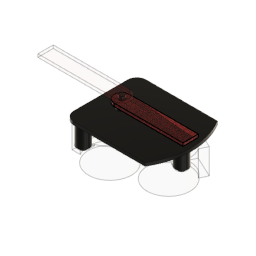
Clock_Assembly (1) (Autodesk Fusion 360 archive; units mm, degrees)
design "Movement"
description: Spur Gear; Module: 1.000000; Num Teeth: 20; Pressure Angle: 20.000000; Backlash: 0.10 mm
Autodesk Fusion 360 part; units mm, degrees
cylinder "CylinderPrimitive1" add diameter 28 height 19 placed x (1, 0, 0) y (0, 1, 0) z (0, 0, 1) at (0, 0, 0) makes body 1 in component "Motor"
sketch "Sketch2" plane through (0, 0, 19) normal (0, 0, 1) x (-1, 0, 0) in component "Motor"
  circle A0 centre (0, 0) radius 14
  line L0 (3.5, -13.5554) -> (3.5, -17.5)
  line L1 (-3.5, -13.5554) -> (-3.5, -17.5)
  line L2 (0, 0) -> (0, -14) construction
  line L3 (3.5, -17.5) -> (-3.5, -17.5) construction
  arc A1 (-3.5, -17.5) -> (3.5, -17.5) centre (0, -17.5) ccw
  circle A2 centre (0, -17.5) radius 2.05
  line L4 (0, 0) -> (-14, 0) construction
  arc A3 (3.5, 17.5) -> (-3.5, 17.5) centre (0, 17.5) ccw
  circle A4 centre (0, 17.5) radius 2.05
  line L5 (3.5, 13.5554) -> (3.5, 17.5)
  line L6 (-3.5, 13.5554) -> (-3.5, 17.5)
  circle A5 centre (-7.8, 0) radius 4.5
  circle A6 centre (-7.8, 0) radius 2.45
  line L7 (-7.8, 0) -> (-7.8, -2.45) construction
  line L8 (-9.3, -1.9371) -> (-9.3, 1.9371)
  line L9 (-6.3, -1.9371) -> (-6.3, 1.9371)
  line L10 (11.8216, -7.5) -> (17.2, -7.5)
  line L11 (17.2, -7.5) -> (17.2, 7.5)
  line L12 (17.2, 7.5) -> (11.8216, 7.5)
  line L13 (14, 0) -> (17.2, 0) construction
  dimension "d3" = 3.5
  dimension "d4" = 3.5
  dimension "d5" = 7
  dimension "d6" = 4.1
  dimension "d7" = 9
  dimension "d9" = 1.7
  dimension "d10" = 4.9
  dimension "d11" = 1.5
  dimension "d12" = 1.5
  dimension "d23" = 7.5
  dimension "d24" = 7.5
  dimension "d25" = 3.2
  constraint coincident A0 L0.start
  constraint vertical L0
  constraint coincident A0 L1.start
  constraint vertical L1
  constraint coincident A0.centre L2.start
  constraint coincident A0 L2.end
  constraint vertical L2
  constraint horizontal L3
  constraint midpoint L3 A1.centre
  constraint concentric A1 A2
  constraint coincident A0 L4.end
  constraint perpendicular L2 L4
  constraint symmetric L0.start L4 L5.start
  constraint symmetric L0.end L4 A3.start
  constraint symmetric L1.start L4 L6.start
  constraint symmetric L1.end L4 A3.end
  constraint symmetric A1 L4 A3
  constraint symmetric A2 L4 A4
  constraint coincident L4 A5.centre
  constraint concentric A5 A6
  constraint coincident A5.centre A6.centre
  constraint coincident A6 L7.end
  constraint perpendicular L4 L7
  constraint coincident A6 L8.start
  constraint coincident A6 L8.end
  constraint vertical L8
  constraint coincident A6 L9.start
  constraint coincident A6 L9.end
  constraint parallel L8 L9
  constraint coincident A0 L10.start
  constraint horizontal L10
  constraint perpendicular L10 L11
  constraint coincident A0 L12.end
  constraint perpendicular L11 L12
  constraint coincident A0 L13.start
  constraint coincident L11 L13.end
  constraint perpendicular L11 L13
  constraint collinear L4 L13
  measures "d3" distance of L0 L2
  measures "d4" distance of L1 L2
  measures "d5" distance of L2.end A1
  measures "d6" diameter of A2
  measures "d7" diameter of A5
  measures "d9" distance of L4.end A5
  measures "d10" diameter of A6
  measures "d11" distance of L7 L8
  measures "d12" distance of L7 L9
  measures "d23" distance of L12 L13
  measures "d24" distance of L10 L13
  measures "d25" distance of A0 L11
extrude "Extrude1" add sketch "Sketch2" against normal blind 0.85 contours A0 A3 L5 L6 | A0 L0 L1 A1 bodies 1 in component "Motor"
extrude "Extrude2" add sketch "Sketch2" along normal blind 1.7 contours A5 | A6 L9 | A6 L8 L9 | A6 L8 bodies 1 in component "Motor"
extrude "Extrude3" add sketch "Sketch2" along normal blind 2.25 from surface at 1.7 contours A6 L9 | A6 L8 L9 | A6 L8 bodies 1 in component "Motor"
extrude "Extrude4" add sketch "Sketch2" along normal blind 10 contours A6 L8 L9 bodies 1 in component "Motor"
extrude "Extrude5" add sketch "Sketch2" against normal blind 16.5 contours A0 L10 L11 L12 bodies 1 in component "Motor"
sketch "Sketch1" plane through (0, 0, 29) normal (0, 0, 1) x (-1, 0, 0) in component "Minute Hand"
  arc A0 (-9.3, -1.9371) -> (-6.3, -1.9371) centre (-7.8, 0) ccw construction
  line L0 (-6.3, -1.9371) -> (-6.3, 1.9371) construction
  arc A1 (-6.3, 1.9371) -> (-9.3, 1.9371) centre (-7.8, 0) ccw construction
  line L1 (-9.3, 1.9371) -> (-9.3, -1.9371)
  line L2 (-6.3, 1.9371) -> (-6.3, -1.9371) construction
  arc A2 (-6.3, -1.9371) -> (-6.3, 1.9371) centre (-7.8, 0) ccw construction
  line L3 (-9.3, -1.9371) -> (-9.3, 1.9371) construction
  arc A3 (-9.3, 1.9371) -> (-9.3, -1.9371) centre (-7.8, 0) ccw construction
  arc A4 (-5.0755, -3.5185) -> (-5.0755, 3.5185) centre (-7.8, 0) ccw
  arc A5 (-5.0755, 3.5185) -> (-10.5245, 3.5185) centre (-7.8, 0) ccw
  arc A6 (-10.5245, 3.5185) -> (-10.5245, -3.5185) centre (-7.8, 0) ccw
  arc A7 (-10.5245, -3.5185) -> (-5.0755, -3.5185) centre (-7.8, 0) ccw
  arc A8 (-6.2, 1.9856) -> (-9.4, 1.9856) centre (-7.8, 0) ccw
  line L4 (-9.4, -1.9856) -> (-9.4, 1.9856)
  arc A9 (-9.4, -1.9856) -> (-6.2, -1.9856) centre (-7.8, 0) ccw
  line L5 (-6.2, -1.9856) -> (-6.2, 1.9856)
  circle A10 centre (-7.8, 0) radius 1.6
  dimension "d28" = 2
  dimension "d29" = 0.1
  dimension "d32" = 3.2
  constraint concentric A3 A10
  measures "d32" diameter of A10
extrude "Extrude1'" add sketch "Sketch1" against normal up to surface (5.05 mm away) separate body makes body 2 in component "Minute Hand"
extrude "Extrude3'" add sketch "Sketch1" along normal blind 1 contours L1 A10 | A8 L4 L5 A10 | L1 A10 | L4 A9 L5 A10 | A4 A5 A6 A7 bodies 2 in component "Minute Hand"
extrude "Extrude2'" add sketch "Sketch1" along normal blind 12.5 from surface at 1 contours L1 A10 | L1 A10 bodies 2 in component "Minute Hand"
sketch "Sketch1 (2)" plane through (0, 0, 0) normal (0, 0, 1) x (1, 0, 0) in component "Hour Hand"
  circle A0 centre (0, 0) radius 8.7492
extrude "Extrude1''" add sketch "Sketch1 (2)" along normal blind 3 separate body makes body 3 in component "Hour Hand"
sketch "Sketch2 (2)" plane through (0, 0, 0) normal (0, 0, 1) x (1, 0, 0) in component "Hour Hand"
  spline S0 degree 5 poles (9.3581, -0.8534) (9.3628, -0.8538) (9.3721, -0.8546) (9.3861, -0.8553) (9.4048, -0.8555) (9.4282, -0.8549) (9.4516, -0.8535) (9.4751, -0.8518) (9.4986, -0.8498) (9.5221, -0.8476) (9.5456, -0.8452) (9.5692, -0.8427) (9.5927, -0.8398) (9.6163, -0.8366) (9.6398, -0.8331) (9.6634, -0.8293) (9.687, -0.8252) (9.7106, -0.8208) (9.7342, -0.8163) (9.7577, -0.8116) (9.7813, -0.8067) (9.8049, -0.8015) (9.8285, -0.7962) (9.8521, -0.7907) (9.8757, -0.7849) (9.8993, -0.779) (9.9228, -0.7729) (9.9464, -0.7665) (9.97, -0.76) (9.9935, -0.7533) (10.0171, -0.7465) (10.0407, -0.7394) (10.0642, -0.7322) (10.0877, -0.7249) (10.1113, -0.7173) (10.1348, -0.7096) (10.1583, -0.7017) (10.1818, -0.6937) (10.2053, -0.6855) (10.2288, -0.6771) (10.2523, -0.6686) (10.2758, -0.6599) (10.2992, -0.6511) (10.3227, -0.6421) (10.3461, -0.633) (10.3695, -0.6237) (10.3929, -0.6143) (10.4163, -0.6047) (10.4397, -0.5949) (10.463, -0.5851) (10.4864, -0.5751) (10.5097, -0.5649) (10.533, -0.5546) (10.5563, -0.5441) (10.5796, -0.5336) (10.6029, -0.5228) (10.6261, -0.512) (10.6493, -0.501) (10.6726, -0.4898) (10.6957, -0.4785) (10.7189, -0.4671) (10.7421, -0.4556) (10.7652, -0.4439) (10.7883, -0.4321) (10.8114, -0.4201) (10.8345, -0.4081) (10.8575, -0.3959) (10.8806, -0.3835) (10.9036, -0.3711) (10.9265, -0.3585) (10.9495, -0.3458) (10.9679, -0.3355) (10.9816, -0.3277) (10.9908, -0.3225) (10.9953, -0.3199) knots 0 0 0 0 0 0 0.01428571 0.02857143 0.04285714 0.05714286 0.07142857 0.08571429 0.1 0.11428571 0.12857143 0.14285714 0.15714286 0.17142857 0.18571429 0.2 0.21428571 0.22857143 0.24285714 0.25714286 0.27142857 0.28571429 0.3 0.31428571 0.32857143 0.34285714 0.35714286 0.37142857 0.38571429 0.4 0.41428571 0.42857143 0.44285714 0.45714286 0.47142857 0.48571429 0.5 0.51428571 0.52857143 0.54285714 0.55714286 0.57142857 0.58571429 0.6 0.61428571 0.62857143 0.64285714 0.65714286 0.67142857 0.68571429 0.7 0.71428571 0.72857143 0.74285714 0.75714286 0.77142857 0.78571429 0.8 0.81428571 0.82857143 0.84285714 0.85714286 0.87142857 0.88571429 0.9 0.91428571 0.92857143 0.94285714 0.95714286 0.97142857 0.98571429 1 1 1 1 1 1
  spline S1 degree 5 poles (9.3581, 0.8534) (9.3628, 0.8538) (9.3721, 0.8546) (9.3861, 0.8553) (9.4048, 0.8555) (9.4282, 0.8549) (9.4516, 0.8535) (9.4751, 0.8518) (9.4986, 0.8498) (9.5221, 0.8476) (9.5456, 0.8452) (9.5692, 0.8427) (9.5927, 0.8398) (9.6163, 0.8366) (9.6398, 0.8331) (9.6634, 0.8293) (9.687, 0.8252) (9.7106, 0.8208) (9.7342, 0.8163) (9.7577, 0.8116) (9.7813, 0.8067) (9.8049, 0.8015) (9.8285, 0.7962) (9.8521, 0.7907) (9.8757, 0.7849) (9.8993, 0.779) (9.9228, 0.7729) (9.9464, 0.7665) (9.97, 0.76) (9.9935, 0.7533) (10.0171, 0.7465) (10.0407, 0.7394) (10.0642, 0.7322) (10.0877, 0.7249) (10.1113, 0.7173) (10.1348, 0.7096) (10.1583, 0.7017) (10.1818, 0.6937) (10.2053, 0.6855) (10.2288, 0.6771) (10.2523, 0.6686) (10.2758, 0.6599) (10.2992, 0.6511) (10.3227, 0.6421) (10.3461, 0.633) (10.3695, 0.6237) (10.3929, 0.6143) (10.4163, 0.6047) (10.4397, 0.5949) (10.463, 0.5851) (10.4864, 0.5751) (10.5097, 0.5649) (10.533, 0.5546) (10.5563, 0.5441) (10.5796, 0.5336) (10.6029, 0.5228) (10.6261, 0.512) (10.6493, 0.501) (10.6726, 0.4898) (10.6957, 0.4785) (10.7189, 0.4671) (10.7421, 0.4556) (10.7652, 0.4439) (10.7883, 0.4321) (10.8114, 0.4201) (10.8345, 0.4081) (10.8575, 0.3959) (10.8806, 0.3835) (10.9036, 0.3711) (10.9265, 0.3585) (10.9495, 0.3458) (10.9679, 0.3355) (10.9816, 0.3277) (10.9908, 0.3225) (10.9953, 0.3199) knots 0 0 0 0 0 0 0.01428571 0.02857143 0.04285714 0.05714286 0.07142857 0.08571429 0.1 0.11428571 0.12857143 0.14285714 0.15714286 0.17142857 0.18571429 0.2 0.21428571 0.22857143 0.24285714 0.25714286 0.27142857 0.28571429 0.3 0.31428571 0.32857143 0.34285714 0.35714286 0.37142857 0.38571429 0.4 0.41428571 0.42857143 0.44285714 0.45714286 0.47142857 0.48571429 0.5 0.51428571 0.52857143 0.54285714 0.55714286 0.57142857 0.58571429 0.6 0.61428571 0.62857143 0.64285714 0.65714286 0.67142857 0.68571429 0.7 0.71428571 0.72857143 0.74285714 0.75714286 0.77142857 0.78571429 0.8 0.81428571 0.82857143 0.84285714 0.85714286 0.87142857 0.88571429 0.9 0.91428571 0.92857143 0.94285714 0.95714286 0.97142857 0.98571429 1 1 1 1 1 1
  arc A0 (10.9953, -0.3199) -> (10.9953, 0.3199) centre (0, 0) ccw
  line L0 (8.7031, -0.7946) -> (9.3581, -0.8534)
  line L1 (8.7031, 0.7946) -> (9.3581, 0.8534)
  line L2 (8.7031, -0.7946) -> (8.7031, 0.7946)
  point P0 (9.4732, -0.8519)
  point P1 (9.5892, -0.8402)
  point P2 (9.7057, -0.8217)
  point P3 (9.8226, -0.7975)
  point P4 (9.9398, -0.7683)
  point P5 (10.0572, -0.7344)
  point P6 (10.1747, -0.6961)
  point P7 (10.2922, -0.6537)
  point P8 (10.4098, -0.6073)
  point P9 (10.5272, -0.5571)
  point P10 (10.6446, -0.5032)
  point P11 (10.7618, -0.4456)
  point P12 (10.8787, -0.3845)
  point P13 (9.4732, 0.8519)
  point P14 (9.5892, 0.8402)
  point P15 (9.7057, 0.8217)
  point P16 (9.8226, 0.7975)
  point P17 (9.9398, 0.7683)
  point P18 (10.0572, 0.7344)
  point P19 (10.1747, 0.6961)
  point P20 (10.2922, 0.6537)
  point P21 (10.4098, 0.6073)
  point P22 (10.5272, 0.5571)
  point P23 (10.6446, 0.5032)
  point P24 (10.7618, 0.4456)
  point P25 (10.8787, 0.3845)
extrude "Extrude2''" add sketch "Sketch2 (2)" along normal blind 3 bodies 3 in component "Hour Hand"
fillet "Fillet1" radius 0.5 2 edges at (8.713, -0.7955, 1.5) (8.713, 0.7955, 1.5) on bodies 3 in component "Hour Hand"
pattern_circular "C-Pattern1" count 20 over 360 about axis through (0, 0, 0) along (0, 0, 1) of "Extrude2''", "Fillet1" in component "Hour Hand"
sketch "Sketch3" plane through (0, 0, 0) normal (0, 0, 1) x (1, 0, 0) in component "Hour Hand"
  circle A0 centre (0, 0) radius 10 construction
sketch "Sketch4" plane through (0, 0, 3) normal (0, 0, 1) x (-1, 0, 0) in component "Hour Hand"
  circle A0 centre (0, 0) radius 1.75
  circle A1 centre (0, 0) radius 3
  dimension "d56" = 3.5
  dimension "d57" = 6
  constraint coincident A0.centre A1.centre
  measures "d56" diameter of A0
  measures "d57" diameter of A1
extrude "Extrude3''" cut sketch "Sketch4" against normal through all contours A0 bodies 3 in component "Hour Hand"
extrude "Extrude4'" add sketch "Sketch4" along normal blind 6.5 bodies 3 in component "Hour Hand"
sketch "Sketch1 (3)" plane through (0, 0, 0) normal (0, 0, 1) x (1, 0, 0) in component "Spur Gear (20 teeth)"
  circle A0 centre (0, 0) radius 8.7492
extrude "Extrude1'''" add sketch "Sketch1 (3)" along normal blind 3 separate body makes body 4 in component "Spur Gear (20 teeth)"
sketch "Sketch2 (3)" plane through (0, 0, 0) normal (0, 0, 1) x (1, 0, 0) in component "Spur Gear (20 teeth)"
  spline S0 degree 5 poles (9.3581, -0.8534) (9.3628, -0.8538) (9.3721, -0.8546) (9.3861, -0.8553) (9.4048, -0.8555) (9.4282, -0.8549) (9.4516, -0.8535) (9.4751, -0.8518) (9.4986, -0.8498) (9.5221, -0.8476) (9.5456, -0.8452) (9.5692, -0.8427) (9.5927, -0.8398) (9.6163, -0.8366) (9.6398, -0.8331) (9.6634, -0.8293) (9.687, -0.8252) (9.7106, -0.8208) (9.7342, -0.8163) (9.7577, -0.8116) (9.7813, -0.8067) (9.8049, -0.8015) (9.8285, -0.7962) (9.8521, -0.7907) (9.8757, -0.7849) (9.8993, -0.779) (9.9228, -0.7729) (9.9464, -0.7665) (9.97, -0.76) (9.9935, -0.7533) (10.0171, -0.7465) (10.0407, -0.7394) (10.0642, -0.7322) (10.0877, -0.7249) (10.1113, -0.7173) (10.1348, -0.7096) (10.1583, -0.7017) (10.1818, -0.6937) (10.2053, -0.6855) (10.2288, -0.6771) (10.2523, -0.6686) (10.2758, -0.6599) (10.2992, -0.6511) (10.3227, -0.6421) (10.3461, -0.633) (10.3695, -0.6237) (10.3929, -0.6143) (10.4163, -0.6047) (10.4397, -0.5949) (10.463, -0.5851) (10.4864, -0.5751) (10.5097, -0.5649) (10.533, -0.5546) (10.5563, -0.5441) (10.5796, -0.5336) (10.6029, -0.5228) (10.6261, -0.512) (10.6493, -0.501) (10.6726, -0.4898) (10.6957, -0.4785) (10.7189, -0.4671) (10.7421, -0.4556) (10.7652, -0.4439) (10.7883, -0.4321) (10.8114, -0.4201) (10.8345, -0.4081) (10.8575, -0.3959) (10.8806, -0.3835) (10.9036, -0.3711) (10.9265, -0.3585) (10.9495, -0.3458) (10.9679, -0.3355) (10.9816, -0.3277) (10.9908, -0.3225) (10.9953, -0.3199) knots 0 0 0 0 0 0 0.01428571 0.02857143 0.04285714 0.05714286 0.07142857 0.08571429 0.1 0.11428571 0.12857143 0.14285714 0.15714286 0.17142857 0.18571429 0.2 0.21428571 0.22857143 0.24285714 0.25714286 0.27142857 0.28571429 0.3 0.31428571 0.32857143 0.34285714 0.35714286 0.37142857 0.38571429 0.4 0.41428571 0.42857143 0.44285714 0.45714286 0.47142857 0.48571429 0.5 0.51428571 0.52857143 0.54285714 0.55714286 0.57142857 0.58571429 0.6 0.61428571 0.62857143 0.64285714 0.65714286 0.67142857 0.68571429 0.7 0.71428571 0.72857143 0.74285714 0.75714286 0.77142857 0.78571429 0.8 0.81428571 0.82857143 0.84285714 0.85714286 0.87142857 0.88571429 0.9 0.91428571 0.92857143 0.94285714 0.95714286 0.97142857 0.98571429 1 1 1 1 1 1
  spline S1 degree 5 poles (9.3581, 0.8534) (9.3628, 0.8538) (9.3721, 0.8546) (9.3861, 0.8553) (9.4048, 0.8555) (9.4282, 0.8549) (9.4516, 0.8535) (9.4751, 0.8518) (9.4986, 0.8498) (9.5221, 0.8476) (9.5456, 0.8452) (9.5692, 0.8427) (9.5927, 0.8398) (9.6163, 0.8366) (9.6398, 0.8331) (9.6634, 0.8293) (9.687, 0.8252) (9.7106, 0.8208) (9.7342, 0.8163) (9.7577, 0.8116) (9.7813, 0.8067) (9.8049, 0.8015) (9.8285, 0.7962) (9.8521, 0.7907) (9.8757, 0.7849) (9.8993, 0.779) (9.9228, 0.7729) (9.9464, 0.7665) (9.97, 0.76) (9.9935, 0.7533) (10.0171, 0.7465) (10.0407, 0.7394) (10.0642, 0.7322) (10.0877, 0.7249) (10.1113, 0.7173) (10.1348, 0.7096) (10.1583, 0.7017) (10.1818, 0.6937) (10.2053, 0.6855) (10.2288, 0.6771) (10.2523, 0.6686) (10.2758, 0.6599) (10.2992, 0.6511) (10.3227, 0.6421) (10.3461, 0.633) (10.3695, 0.6237) (10.3929, 0.6143) (10.4163, 0.6047) (10.4397, 0.5949) (10.463, 0.5851) (10.4864, 0.5751) (10.5097, 0.5649) (10.533, 0.5546) (10.5563, 0.5441) (10.5796, 0.5336) (10.6029, 0.5228) (10.6261, 0.512) (10.6493, 0.501) (10.6726, 0.4898) (10.6957, 0.4785) (10.7189, 0.4671) (10.7421, 0.4556) (10.7652, 0.4439) (10.7883, 0.4321) (10.8114, 0.4201) (10.8345, 0.4081) (10.8575, 0.3959) (10.8806, 0.3835) (10.9036, 0.3711) (10.9265, 0.3585) (10.9495, 0.3458) (10.9679, 0.3355) (10.9816, 0.3277) (10.9908, 0.3225) (10.9953, 0.3199) knots 0 0 0 0 0 0 0.01428571 0.02857143 0.04285714 0.05714286 0.07142857 0.08571429 0.1 0.11428571 0.12857143 0.14285714 0.15714286 0.17142857 0.18571429 0.2 0.21428571 0.22857143 0.24285714 0.25714286 0.27142857 0.28571429 0.3 0.31428571 0.32857143 0.34285714 0.35714286 0.37142857 0.38571429 0.4 0.41428571 0.42857143 0.44285714 0.45714286 0.47142857 0.48571429 0.5 0.51428571 0.52857143 0.54285714 0.55714286 0.57142857 0.58571429 0.6 0.61428571 0.62857143 0.64285714 0.65714286 0.67142857 0.68571429 0.7 0.71428571 0.72857143 0.74285714 0.75714286 0.77142857 0.78571429 0.8 0.81428571 0.82857143 0.84285714 0.85714286 0.87142857 0.88571429 0.9 0.91428571 0.92857143 0.94285714 0.95714286 0.97142857 0.98571429 1 1 1 1 1 1
  arc A0 (10.9953, -0.3199) -> (10.9953, 0.3199) centre (0, 0) ccw
  line L0 (8.7031, -0.7946) -> (9.3581, -0.8534)
  line L1 (8.7031, 0.7946) -> (9.3581, 0.8534)
  line L2 (8.7031, -0.7946) -> (8.7031, 0.7946)
  point P0 (9.4732, -0.8519)
  point P1 (9.5892, -0.8402)
  point P2 (9.7057, -0.8217)
  point P3 (9.8226, -0.7975)
  point P4 (9.9398, -0.7683)
  point P5 (10.0572, -0.7344)
  point P6 (10.1747, -0.6961)
  point P7 (10.2922, -0.6537)
  point P8 (10.4098, -0.6073)
  point P9 (10.5272, -0.5571)
  point P10 (10.6446, -0.5032)
  point P11 (10.7618, -0.4456)
  point P12 (10.8787, -0.3845)
  point P13 (9.4732, 0.8519)
  point P14 (9.5892, 0.8402)
  point P15 (9.7057, 0.8217)
  point P16 (9.8226, 0.7975)
  point P17 (9.9398, 0.7683)
  point P18 (10.0572, 0.7344)
  point P19 (10.1747, 0.6961)
  point P20 (10.2922, 0.6537)
  point P21 (10.4098, 0.6073)
  point P22 (10.5272, 0.5571)
  point P23 (10.6446, 0.5032)
  point P24 (10.7618, 0.4456)
  point P25 (10.8787, 0.3845)
extrude "Extrude2'''" add sketch "Sketch2 (3)" along normal blind 3 bodies 4 in component "Spur Gear (20 teeth)"
fillet "Fillet1'" radius 0.5 2 edges at (8.713, -0.7955, 1.5) (8.713, 0.7955, 1.5) on bodies 4 in component "Spur Gear (20 teeth)"
pattern_circular "C-Pattern1'" count 20 over 360 about axis through (0, 0, 0) along (0, 0, 1) of "Extrude2'''", "Fillet1'" in component "Spur Gear (20 teeth)"
sketch "Sketch3 (2)" plane through (0, 0, 0) normal (0, 0, 1) x (1, 0, 0) in component "Spur Gear (20 teeth)"
  circle A0 centre (0, 0) radius 10 construction
sketch "Sketch4 (2)" plane through (0, 0, 3) normal (0, 0, 1) x (-1, 0, 0) in component "Spur Gear (20 teeth)"
  arc A0 (2.3896, -0.5408) -> (1.1217, 2.1781) centre (0, 0) ccw construction
  line L0 (2.3896, -0.5408) -> (-1.1217, -2.1781) construction
  arc A1 (-2.3896, 0.5408) -> (-1.1217, -2.1781) centre (0, 0) ccw construction
  line L1 (-2.3896, 0.5408) -> (1.1217, 2.1781) construction
  arc A2 (1.1217, 2.1781) -> (-2.3896, 0.5408) centre (0, 0) ccw construction
  arc A3 (-1.1217, -2.1781) -> (2.3896, -0.5408) centre (0, 0) ccw construction
  arc A4 (2.0374, 3.9562) -> (-4.3402, 0.9823) centre (0, 0) ccw
  arc A5 (-4.3402, 0.9823) -> (-2.0374, -3.9562) centre (0, 0) ccw
  arc A6 (-2.0374, -3.9562) -> (4.3402, -0.9823) centre (0, 0) ccw
  arc A7 (4.3402, -0.9823) -> (2.0374, 3.9562) centre (0, 0) ccw
  line L2 (-2.4757, 0.611) -> (1.1234, 2.2892)
  arc A8 (2.4757, -0.611) -> (1.1234, 2.2892) centre (0, 0) ccw
  line L3 (2.4757, -0.611) -> (-1.1234, -2.2892)
  arc A9 (-2.4757, 0.611) -> (-1.1234, -2.2892) centre (0, 0) ccw
  dimension "d70" = 2
  dimension "d71" = 0.1
extrude "Extrude3'''" add sketch "Sketch4 (2)" along normal up to surface (3.05 mm away) bodies 4 in component "Spur Gear (20 teeth)"
extrude "Extrude4''" cut sketch "Sketch4 (2)" against normal up to surface (2 mm away) contours L2 A8 L3 A9 bodies 4 in component "Spur Gear (20 teeth)"
sketch "Sketch2 (4)" plane through (0, 0, 2) normal (0, 0, 1) x (-1, 0, 0) in component "Face"
  line L0 (-38.6174, -23.55) -> (13.85, -23.55)
  line L1 (13.85, -23.55) -> (13.85, 23.55)
  line L2 (13.85, 23.55) -> (-38.6174, 23.55)
  line L3 (-12.5139, -15.9701) -> (-8.9389, -17.6371)
  line L4 (11.3, -13.5554) -> (11.3, -17.5)
  line L5 (0, 0) -> (-15.4197, 0) construction
  circle A0 centre (-7.4598, -14.465) radius 2.05 construction
  circle A1 centre (-39.1805, 0.3266) radius 2.05 construction
  circle A2 centre (7.8, 17.5) radius 2.05 construction
  circle A3 centre (7.8, -17.5) radius 2.05 construction
  circle A4 centre (0, 0) radius 3 construction
  circle A5 centre (7.8, 17.5) radius 1.95
  circle A6 centre (-39.1805, 0.3266) radius 1.95
  circle A7 centre (7.8, -17.5) radius 1.95
  circle A8 centre (-7.4598, -14.465) radius 1.95
  circle A9 centre (7.8, 17.5) radius 4.05
  circle A10 centre (-39.1805, 0.3266) radius 4.05
  circle A11 centre (-7.4598, -14.465) radius 4.05
  circle A12 centre (7.8, -17.5) radius 4.05
  circle A13 centre (0, 0) radius 3.2
  line L6 (-43.2305, 5.0074) -> (-43.2305, 0.3266) construction
  line L7 (11.85, -17.5) -> (13.85, -17.5) construction
  line L8 (11.85, -17.5) -> (11.85, -15.2011) construction
  line L9 (7.8, -21.55) -> (7.8, -23.55) construction
  line L10 (7.8, -21.55) -> (5.4417, -21.55) construction
  line L11 (7.8, 21.55) -> (7.8, 23.55) construction
  line L12 (7.8, 21.55) -> (6.3222, 21.55) construction
  arc A14 (-38.6174, 23.55) -> (-38.6174, -23.55) centre (0, 0) ccw
  line L13 (-45.2305, 0.3266) -> (-43.2305, 0.3266) construction
  point P0 (-15.4197, 0)
  dimension "d81" = -0.1
  dimension "d82" = -0.1
  dimension "d83" = -0.1
  dimension "d84" = -0.1
  dimension "d85" = 2
  dimension "d86" = 2
  dimension "d87" = 2
  dimension "d88" = 2
  dimension "d89" = 0.2
  dimension "d102" = 2
  constraint horizontal L0
  constraint perpendicular L0 L1
  constraint parallel L0 L2
  constraint coincident L5.start A4.centre
  constraint coincident P0 L5.end
  constraint horizontal L5
  constraint coincident A10 L6.end
  constraint tangent A10 L6
  constraint vertical L6
  constraint coincident A12 L7.start
  constraint coincident L1 L7.end
  constraint perpendicular L1 L7
  constraint perpendicular L7 L8
  constraint tangent A12 L8
  constraint coincident A12 L9.start
  constraint coincident L0 L9.end
  constraint perpendicular L0 L9
  constraint perpendicular L9 L10
  constraint tangent A12 L10
  constraint coincident A9 L11.start
  constraint coincident L2 L11.end
  constraint perpendicular L2 L11
  constraint perpendicular L11 L12
  constraint tangent A9 L12
  constraint equal L7 L11
  constraint equal L7 L9
  constraint coincident L0 A14.end
  constraint coincident L2 A14.start
  constraint coincident A14 L13.start
  constraint equal L9 L13
  constraint horizontal L13
  measures "d102" distance of L6.end L13.start
extrude "Extrude1''''" add sketch "Sketch2 (4)" along normal blind 2 separate body contours L0 L1 L2 A14 | A5 | A6 | A7 | A8 | A9 | A10 | A11 | A12 | A13 makes body 5 in component "Face"
extrude "Extrude2''''" add sketch "Sketch2 (4)" against normal up to surface (14 mm away) contours A9 | A12 bodies 5 in component "Face"
extrude "Extrude3''''" add sketch "Sketch2 (4)" against normal up to surface (16 mm away) contours A5 | A7 bodies 5 in component "Face"
extrude "Extrude4'''" add sketch "Sketch2 (4)" against normal up to surface (11 mm away) contours A10 | A11 bodies 5 in component "Face"
extrude "Extrude5'" add sketch "Sketch2 (4)" against normal up to surface (13 mm away) contours A6 | A8 bodies 5 in component "Face"
extrude "Extrude6" cut sketch "Sketch2 (4)" along normal through all contours A13 bodies 5 in component "Face"
fillet "Fillet1''" radius 6 2 edges at (-13.85, -23.55, 3) (-13.85, 23.55, 3) on bodies 5 in component "Face"
sketch "Sketch1 (4)" plane through (0, 0, 8.5) normal (0, 0, 1) x (-1, 0, 0) in component "Hour Hand (1)"
  circle A0 centre (0, 0) radius 1.75
  circle A1 centre (0, 0) radius 3 construction
  arc A2 (0, -5) -> (0, 5) centre (0, 0) ccw
  line L0 (0, -5) -> (-44.7214, -5)
  line L1 (-44.7214, -5) -> (-44.7214, 5)
  line L2 (-44.7214, 5) -> (0, 5)
  circle A3 centre (0, 0) radius 45 construction
  circle A4 centre (0, 0) radius 3.01
  dimension "d103" = 5
  dimension "d104" = 90
  dimension "d105" = 0.01
  constraint coincident A0.centre A1.centre
  constraint tangent A2 L0
  constraint horizontal L0
  constraint perpendicular L0 L1
  constraint tangent A2 L2
  constraint coincident L1.end A3
  measures "d103" radius of A2
  measures "d104" diameter of A3
extrude "Extrude1'''''" add sketch "Sketch1 (4)" against normal blind 1.5 separate body contours A2 L0 L1 L2 makes body 6 in component "Hour Hand (1)"
extrude "Extrude2'''''" add sketch "Sketch1 (4)" along normal blind 0.5 contours A2 L0 L1 L2 | A4 bodies 6 in component "Hour Hand (1)"
sketch "Sketch1 (5)" plane through (0, 0, 11.5) normal (0, 0, 1) x (-1, 0, 0) in component "Minute Hand (1)"
  circle A0 centre (0, 0) radius 1.6 construction
  circle A1 centre (0, 0) radius 1.7
  arc A2 (0, 5) -> (0, -5) centre (0, 0) ccw
  circle A3 centre (0, 0) radius 50 construction
  line L0 (0, -5) -> (49.7494, -5)
  line L1 (49.7494, -5) -> (49.7494, 5)
  line L2 (0, 5) -> (49.7494, 5)
  dimension "d110" = 0.1
  dimension "d111" = 5
  dimension "d112" = 100
  constraint coincident A0.centre A1.centre
  constraint concentric A0 A3
  constraint coincident A3 L0.end
  constraint tangent A2 L0
  constraint horizontal L0
  constraint coincident A3 L1.end
  constraint perpendicular L0 L1
  constraint tangent A2 L2
  measures "d111" radius of A2
  measures "d112" diameter of A3
extrude "Extrude1''''''" add sketch "Sketch1 (5)" along normal blind 0.5 separate body contours A1 | A2 L0 L1 L2 makes body 7 in component "Minute Hand (1)"
extrude "Extrude2''''''" add sketch "Sketch1 (5)" against normal blind 1.5 bodies 7 in component "Minute Hand (1)"
component "Face" placed x (1, 0, 0) y (0, 1, 0) z (0, 0, 1) at (0, 0, 0)
component "Motor" placed x (1, 0, 0) y (0, 1, 0) z (0, 0, 1) at (-7.8, 0, -31)
component "Minute Hand" placed x (1, 0, 0) y (0, 1, 0) z (0, 0, 1) at (-7.8, 0, -31)
component "Motor" placed x (-0.422618, -0.906308, 0) y (0.906308, -0.422618, 0) z (0, 0, 1) at (23.3201, 7.0692, -28)
component "Hour Hand" placed x (1, 0, 0) y (0, 1, 0) z (0, 0, 1) at (0, 0, -1)
component "Spur Gear (20 teeth)" placed x (-1, 0, 0) y (0, 1, 0) z (0, 0, -1) at (20.0237, 0, 2)
component "Hour Hand (1)" placed x (1, 0, 0) y (0, 1, 0) z (0, 0, 1) at (0, 0, 0)
component "Minute Hand (1)" placed x (1, 0, 0) y (0, 1, 0) z (0, 0, 1) at (0, 0, 0)
equation "d34 = 5 mm + PlateThickness + 1 mm + HandTop + HandShaft + HandShaft + 0.5 mm + 1 mm"
equation "d59 = PlateThickness + 2 mm + HandShaft + 0.5 mm + 1 mm"
equation "PlateThickness = 1.5 mm"
equation "d106 = -HandShaft"
equation "d108 = HandTop"
equation "d113 = HandTop"
equation "d115 = -HandShaft"
equation "HandTop = 0.5 mm"
equation "HandShaft = 1.5 mm"
